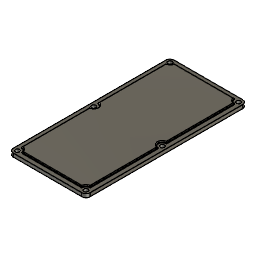
tapa trasera baqueano (Autodesk Fusion 360 design; units mm, degrees)
Autodesk Fusion 360 part; units mm, degrees
sketch "Boceto1" plane through (0, 0, 0) normal (0, 0, 1) x (1, 0, 0)
  circle A0 centre (24.5, 54.5) radius 1.5
  arc A1 (27.5, 54.5) -> (24.5, 57.5) centre (24.5, 54.5) ccw
  arc A2 (-24.5, -3) -> (-24.5, 3) centre (-24.5, 0) ccw
  line L0 (27.5, -54.5) -> (27.5, 54.5)
  circle A3 centre (-24.5, 0) radius 1.5
  arc A4 (24.5, -57.5) -> (27.5, -54.5) centre (24.5, -54.5) ccw
  line L1 (-24.5, 51.5) -> (-24.5, 3)
  line L2 (21.5, 54.5) -> (-21.5, 54.5)
  arc A5 (24.5, 3) -> (24.5, -3) centre (24.5, 0) ccw
  arc A6 (-27.5, -54.5) -> (-24.5, -57.5) centre (-24.5, -54.5) ccw
  arc A7 (21.5, 54.5) -> (24.5, 51.5) centre (24.5, 54.5) ccw
  line L3 (24.5, 3) -> (24.5, 51.5)
  arc A8 (-27.5, -54.5) -> (-24.5, -57.5) centre (-24.5, -54.5) ccw
  arc A9 (-21.5, -54.5) -> (-24.5, -51.5) centre (-24.5, -54.5) ccw
  arc A10 (24.5, -51.5) -> (21.5, -54.5) centre (24.5, -54.5) ccw
  arc A11 (-24.5, 57.5) -> (-27.5, 54.5) centre (-24.5, 54.5) ccw
  line L4 (-24.5, -57.5) -> (24.5, -57.5)
  circle A12 centre (-24.5, 54.5) radius 1.5
  arc A13 (-24.5, 51.5) -> (-21.5, 54.5) centre (-24.5, 54.5) ccw
  arc A14 (27.5, 54.5) -> (24.5, 57.5) centre (24.5, 54.5) ccw
  arc A15 (24.5, -57.5) -> (27.5, -54.5) centre (24.5, -54.5) ccw
  line L5 (27.5, -57.5) -> (26.9159, -56.2786) construction
  circle A16 centre (24.5, 0) radius 1.5
  circle A17 centre (24.5, -54.5) radius 1.5
  line L6 (-21.5, -54.5) -> (21.5, -54.5)
  line L7 (24.5, 57.5) -> (-24.5, 57.5)
  circle A18 centre (-24.5, -54.5) radius 1.5
  arc A19 (-24.5, 57.5) -> (-27.5, 54.5) centre (-24.5, 54.5) ccw
  line L8 (-24.5, -3) -> (-24.5, -51.5)
  line L9 (-27.5, 54.5) -> (-27.5, -54.5)
  line L10 (-27.5, -57.5) -> (-26.9159, -56.2786) construction
  line L11 (24.5, -51.5) -> (24.5, -3)
  dimension "d1" = 3
  dimension "d2" = 3
  dimension "d3" = 3
  dimension "d4" = 3
  dimension "d5" = 6
  dimension "d6" = 6
  dimension "d7" = 6
  dimension "d8" = 6
  dimension "d9" = 3
  dimension "d10" = 3
  dimension "d11" = 3
  dimension "d12" = 3
  dimension "d13" = 6
  dimension "d14" = 3
  dimension "d15" = 6
  dimension "d16" = 3
  constraint horizontal L4
  constraint perpendicular L0 L4
  constraint parallel L4 L7
  constraint parallel L0 L9
  constraint tangent A11 L7
  constraint tangent A11 L9
  constraint tangent A1 L7
  constraint tangent A1 L0
  constraint coincident L10.start L9
  constraint coincident L10.start L4
  constraint tangent A8 L9
  constraint tangent A8 L4
  constraint coincident L5.start L0
  constraint coincident L5.start L4
  constraint tangent L0 A4
  constraint tangent A4 L4
  constraint concentric A6 A8
  constraint concentric A4 A15
  constraint concentric A11 A19
  constraint concentric A1 A14
  constraint concentric A11 A12
  constraint concentric A0 A1
  constraint concentric A6 A18
  constraint concentric A4 A17
  constraint concentric A6 A9
  constraint concentric A10 A15
  constraint coincident L5.end A4
  constraint coincident L10.end A8
  constraint concentric A7 A14
  constraint concentric A13 A19
  constraint concentric A2 A3
  constraint collinear L1 L8
  constraint coincident A2.centre L8
  constraint concentric A5 A16
  constraint collinear L3 L11
  constraint coincident A5.centre L11
  measures "d1" radius of A11
  measures "d2" radius of A1
  measures "d3" radius of A8
  measures "d4" radius of A4
  measures "d5" diameter of A6
  measures "d6" diameter of A15
  measures "d7" diameter of A19
  measures "d8" diameter of A14
  measures "d9" diameter of A12
  measures "d10" diameter of A0
  measures "d11" diameter of A18
  measures "d12" diameter of A17
  measures "d13" diameter of A2
  measures "d14" diameter of A3
  measures "d15" diameter of A5
  measures "d16" diameter of A16
extrude "Extruir1" add sketch "Boceto1" along normal blind 2 contours A2 L1 L2 A5 A7 L3 A9 A10 A13 L6 L8 L11
extrude "Extruir2" add sketch "Boceto1" along normal blind 1 contours A0 | A1 L0 A4 A6 A8 A11 L4 A14 A15 L7 A19 L9 | A2 L1 L2 A5 A7 L3 A9 A10 A13 L6 L8 L11 | A3 | A12 | A16 | A17 | A18
extrude "Extruir3" add 1 faces at (-7.4865, 35.5549, 2) along direction (0, 0, 1) blind 3
extrude "Extruir4" add 1 faces at (26.5, 1, 1) along direction (0, 0, 1) blind 2
hole "Agujero1" at (-24.5, 0, 3) direction (0, 0, -1) diameter 3 depth 5 tip angle 180
hole "Agujero2" at (24.5, 0, 3) direction (0, 0, -1) diameter 3 depth 5 tip angle 180
hole "Agujero3" at (24.5, 54.5, 3) direction (0, 0, -1) diameter 3 depth 5 tip angle 180
hole "Agujero4" at (-24.5, 54.5, 3) direction (0, 0, -1) diameter 3 depth 5 tip angle 180
hole "Agujero5" at (-24.5, -54.5, 3) direction (0, 0, -1) diameter 3 depth 5 tip angle 180
hole "Agujero6" at (24.5, -54.5, 3) direction (0, 0, -1) diameter 3 depth 5 tip angle 180
extrude "Extruir5" cut 1 faces at (-7.4865, 35.5549, 5) along direction (0, 0, -1) blind 1
fillet "Empalme1" radius 0.5 1 faces at (-7.8207, -18.5837, 0)
fillet "Empalme2" radius 0.5 1 faces at (-7.4865, 35.5549, 4)
